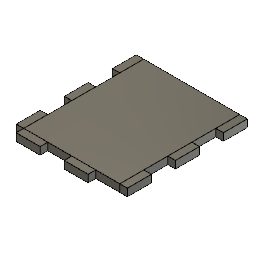
Assembly (Autodesk Fusion 360 archive; units mm, degrees)
design "Top"
Autodesk Fusion 360 part; units mm, degrees
sketch "Sketch1" plane through (0, 0, 0) normal (0, 1, 0) x (1, 0, 0)
  line L0 (0, 0) -> (80, 0)
  line L1 (80, 0) -> (80, 100)
  line L2 (80, 100) -> (0, 100)
  line L3 (0, 100) -> (0, 0)
  line L4 (0, 0) -> (20, 0)
  line L5 (20, 0) -> (20, -6.35)
  line L6 (20, -6.35) -> (0, -6.35)
  line L7 (0, -6.35) -> (0, 0)
  line L8 (40, 0) -> (60, 0)
  line L9 (60, 0) -> (60, -6.35)
  line L10 (60, -6.35) -> (40, -6.35)
  line L11 (40, -6.35) -> (40, 0)
  line L12 (0, 0) -> (-6.35, 0)
  line L13 (-6.35, 0) -> (-6.35, 20)
  line L14 (-6.35, 20) -> (0, 20)
  line L15 (0, 20) -> (0, 0)
  line L16 (0, 40) -> (-6.35, 40)
  line L17 (-6.35, 40) -> (-6.35, 60)
  line L18 (-6.35, 60) -> (0, 60)
  line L19 (0, 60) -> (0, 40)
  line L20 (0, 80) -> (-6.35, 80)
  line L21 (-6.35, 80) -> (-6.35, 100)
  line L22 (-6.35, 100) -> (0, 100)
  line L23 (0, 100) -> (0, 80)
  line L24 (80, 0) -> (86.35, 0)
  line L25 (86.35, 0) -> (86.35, 20)
  line L26 (86.35, 20) -> (80, 20)
  line L27 (80, 20) -> (80, 0)
  line L28 (80, 60) -> (86.35, 60)
  line L29 (86.35, 60) -> (86.35, 40)
  line L30 (86.35, 40) -> (80, 40)
  line L31 (80, 40) -> (80, 60)
  line L32 (80, 100) -> (86.35, 100)
  line L33 (86.35, 100) -> (86.35, 80)
  line L34 (86.35, 80) -> (80, 80)
  line L35 (80, 80) -> (80, 100)
  dimension "d1" = 100
  dimension "d2" = 80
  dimension "d5" = 20
  dimension "d6" = 6.35
  dimension "d7" = 6.35
  dimension "d8" = 20
  dimension "d9" = 20
  dimension "d10" = 6.35
  dimension "d11" = 20
  dimension "d12" = 6.35
  dimension "d13" = 20
  dimension "d14" = 20
  dimension "d15" = 6.35
  dimension "d16" = 20
  dimension "d17" = 20
  dimension "d18" = 6.35
  dimension "d19" = 20
  dimension "d20" = 6.35
  dimension "d21" = 20
  dimension "d22" = 20
  dimension "d23" = 6.35
  dimension "d24" = 20
  measures "d1" distance of L0.start
  measures "d2" distance of L0.start
  measures "d6" distance of L0.start
  measures "d9" distance of L5 L11
  measures "d10" distance of L0.start
  measures "d14" distance of L14 L16
  measures "d17" distance of L18 L20
  measures "d19" distance of L0.start
extrude "Extrude2" add sketch "Sketch1" along normal blind 6.35 makes body 1
extrude "Extrude1" add sketch "Sketch1" along normal blind 6.35 separate body contours L0 L1 L2 L3 L4 L8 L15 L19 L23 L27 L31 L35 makes body 2

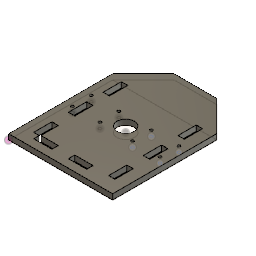
design "Base"
Autodesk Fusion 360 part; units mm, degrees
sketch "Sketch1" plane through (0, 0, 0) normal (0, 1, 0) x (1, 0, 0)
  line L0 (0, 0) -> (120, 0)
  line L1 (120, 0) -> (120, 120)
  line L2 (120, 120) -> (0, 120)
  line L3 (0, 120) -> (0, 0)
  line L4 (0, 120) -> (35.3553, 155.3553)
  line L5 (120, 120) -> (84.6447, 155.3553)
  line L6 (35.3553, 155.3553) -> (84.6447, 155.3553)
  circle A0 centre (60, 75) radius 10
  circle A1 centre (9.5, 64.15) radius 1.65
  circle A2 centre (41.25, 64.15) radius 1.65
  circle A3 centre (41.25, 85.85) radius 1.65
  circle A4 centre (9.5, 85.85) radius 1.65
  circle A5 centre (110.5, 85.85) radius 1.65
  circle A6 centre (110.5, 64.15) radius 1.65
  circle A7 centre (78.75, 64.15) radius 1.65
  circle A8 centre (78.75, 85.85) radius 1.65
  dimension "d1" = 120
  dimension "d2" = 120
  dimension "d3" = 50
  dimension "d4" = 45
  dimension "d5" = 50
  dimension "d6" = 45
  dimension "d7" = 20
  dimension "d8" = 75
  dimension "d9" = 60
  dimension "d10" = 3.3
  dimension "d11" = 3.3
  dimension "d12" = 9.5
  dimension "d13" = 31.75
  dimension "d14" = 10.85
  dimension "d15" = 10.85
  dimension "d16" = 3.3
  dimension "d17" = 3.3
  dimension "d18" = 21.7
  dimension "d19" = 21.7
  dimension "d20" = 9.5
  dimension "d21" = 31.75
  dimension "d22" = 3.3
  dimension "d23" = 3.3
  dimension "d24" = 31.75
  dimension "d25" = 3.3
  dimension "d26" = 3.3
  dimension "d27" = 21.7
  dimension "d28" = 21.7
  dimension "d29" = 31.75
  dimension "d30" = 9.5
  measures "d4" angle of L2 L4
  measures "d6" angle of L2 L5
  measures "d7" diameter of A0
  measures "d10" diameter of A1
  measures "d11" diameter of A2
  measures "d13" distance of L0.start
  measures "d15" distance of L0.start
  measures "d16" diameter of A3
  measures "d17" diameter of A4
  measures "d21" distance of L0.start
  measures "d22" diameter of A7
  measures "d23" diameter of A6
  measures "d25" diameter of A5
  measures "d26" diameter of A8
extrude "Extrude1" add sketch "Sketch1" along normal blind 6.35
sketch "Sketch2" plane through (0, 6.35, 0) normal (0, 1, 0) x (-1, 0, 0)
  circle A0 centre (-78.75, -64.15) radius 1.65
  circle A1 centre (-78.75, -85.85) radius 1.65
  circle A2 centre (-41.25, -85.85) radius 1.65
  circle A3 centre (-9.5, -85.85) radius 1.65
  circle A4 centre (-110.5, -85.85) radius 1.65
  circle A5 centre (-41.25, -64.15) radius 1.65
  circle A6 centre (-9.5, -64.15) radius 1.65
  circle A7 centre (-60, -75) radius 10
  circle A8 centre (-110.5, -64.15) radius 1.65
  line L0 (0, -120) -> (0, 0)
  line L1 (0, 0) -> (-120, 0)
  line L2 (-120, 0) -> (-120, -120)
  line L3 (-120, -120) -> (-84.6447, -155.3553)
  line L4 (-84.6447, -155.3553) -> (-35.3553, -155.3553)
  line L5 (-35.3553, -155.3553) -> (0, -120)
  line L6 (-20, -16.35) -> (-40, -16.35)
  line L7 (-40, -16.35) -> (-40, -10)
  line L8 (-40, -10) -> (-20, -10)
  line L9 (-20, -10) -> (-20, -16.35)
  line L10 (0, 0) -> (-120, 0)
  line L11 (0, -120) -> (0, 0)
  line L12 (-60, -16.35) -> (-80, -16.35)
  line L13 (-80, -16.35) -> (-80, -10)
  line L14 (-80, -10) -> (-60, -10)
  line L15 (-60, -10) -> (-60, -16.35)
  line L16 (-20, -16.35) -> (-13.65, -16.35)
  line L17 (-13.65, -16.35) -> (-13.65, -36.35)
  line L18 (-13.65, -36.35) -> (-20, -36.35)
  line L19 (-20, -36.35) -> (-20, -16.35)
  line L20 (-13.65, -56.35) -> (-20, -56.35)
  line L21 (-20, -56.35) -> (-20, -76.35)
  line L22 (-20, -76.35) -> (-13.65, -76.35)
  line L23 (-13.65, -76.35) -> (-13.65, -56.35)
  line L24 (-20, -96.35) -> (-13.65, -96.35)
  line L25 (-13.65, -96.35) -> (-13.65, -116.35)
  line L26 (-13.65, -116.35) -> (-20, -116.35)
  line L27 (-20, -116.35) -> (-20, -96.35)
  line L28 (-106.35, -16.35) -> (-100, -16.35)
  line L29 (-100, -16.35) -> (-100, -36.35)
  line L30 (-100, -36.35) -> (-106.35, -36.35)
  line L31 (-106.35, -36.35) -> (-106.35, -16.35)
  line L32 (-120, 0) -> (-120, -120)
  line L33 (-100, -76.35) -> (-106.35, -76.35)
  line L34 (-106.35, -76.35) -> (-106.35, -56.35)
  line L35 (-106.35, -56.35) -> (-100, -56.35)
  line L36 (-100, -56.35) -> (-100, -76.35)
  line L37 (-100, -96.35) -> (-106.35, -96.35)
  line L38 (-106.35, -96.35) -> (-106.35, -116.35)
  line L39 (-106.35, -116.35) -> (-100, -116.35)
  line L40 (-100, -116.35) -> (-100, -96.35)
  line L41 (-99.5, -116.85) -> (-99.5, -95.85)
  line L42 (-99.5, -95.85) -> (-106.85, -95.85)
  line L43 (-106.85, -95.85) -> (-106.85, -116.85)
  line L44 (-106.85, -116.85) -> (-99.5, -116.85)
  line L45 (-99.5, -55.85) -> (-99.5, -76.85)
  line L46 (-99.5, -76.85) -> (-106.85, -76.85)
  line L47 (-106.85, -76.85) -> (-106.85, -55.85)
  line L48 (-106.85, -55.85) -> (-99.5, -55.85)
  line L49 (-99.5, -15.85) -> (-99.5, -36.85)
  line L50 (-99.5, -36.85) -> (-106.85, -36.85)
  line L51 (-106.85, -36.85) -> (-106.85, -15.85)
  line L52 (-106.85, -15.85) -> (-99.5, -15.85)
  line L53 (-59.5, -16.85) -> (-80.5, -16.85)
  line L54 (-80.5, -16.85) -> (-80.5, -9.5)
  line L55 (-80.5, -9.5) -> (-59.5, -9.5)
  line L56 (-59.5, -9.5) -> (-59.5, -16.85)
  line L57 (-19.5, -16.85) -> (-40.5, -16.85)
  line L58 (-40.5, -16.85) -> (-40.5, -9.5)
  line L59 (-40.5, -9.5) -> (-19.5, -9.5)
  line L60 (-19.5, -9.5) -> (-19.5, -16.85)
  line L61 (-20.5, -15.85) -> (-13.15, -15.85)
  line L62 (-13.15, -15.85) -> (-13.15, -36.85)
  line L63 (-13.15, -36.85) -> (-20.5, -36.85)
  line L64 (-20.5, -36.85) -> (-20.5, -15.85)
  line L65 (-20.5, -55.85) -> (-20.5, -76.85)
  line L66 (-20.5, -76.85) -> (-13.15, -76.85)
  line L67 (-13.15, -76.85) -> (-13.15, -55.85)
  line L68 (-13.15, -55.85) -> (-20.5, -55.85)
  line L69 (-13.15, -116.85) -> (-20.5, -116.85)
  line L70 (-20.5, -116.85) -> (-20.5, -95.85)
  line L71 (-20.5, -95.85) -> (-13.15, -95.85)
  line L72 (-13.15, -95.85) -> (-13.15, -116.85)
  dimension "d33" = 6.35
  dimension "d34" = 20
  dimension "d35" = 10
  dimension "d37" = 6.35
  dimension "d38" = 20
  dimension "d39" = 20
  dimension "d40" = 10
  dimension "d41" = 20
  dimension "d42" = 6.35
  dimension "d43" = 20
  dimension "d44" = 6.35
  dimension "d45" = 20
  dimension "d48" = 20
  dimension "d49" = 6.35
  dimension "d51" = 20
  dimension "d52" = 20
  dimension "d53" = 6.35
  dimension "d55" = 16.35
  dimension "d56" = 20
  dimension "d57" = 20
  dimension "d58" = 20
  dimension "d59" = 20
  dimension "d60" = 20
  dimension "d61" = 6.35
  dimension "d62" = 20
  dimension "d63" = 20
  dimension "d64" = 20
  dimension "d65" = 6.35
  dimension "d66" = 20
  dimension "d67" = 20
  dimension "d68" = 0.5
  dimension "d69" = -0.5
  dimension "d70" = -0.5
  dimension "d71" = -0.5
  dimension "d72" = -0.5
  dimension "d73" = -0.5
  dimension "d74" = 0.5
  dimension "d75" = -0.5
  measures "d35" distance of L8 L10
  measures "d39" distance of L7 L15
  measures "d40" distance of L10 L14
  measures "d41" distance of L0.end
  measures "d42" distance of L0.end
  measures "d44" distance of L0.end
  measures "d45" distance of L18 L20
  measures "d49" distance of L0.end
  measures "d51" distance of L22 L24
  measures "d52" distance of L0.end
  measures "d55" distance of L10 L28
  measures "d56" distance of L29 L32
  measures "d57" distance of L11 L19
  measures "d58" distance of L11 L21
  measures "d59" distance of L11 L27
  measures "d62" distance of L32 L36
  measures "d63" distance of L30 L35
  measures "d66" distance of L32 L40
  measures "d67" distance of L33 L37
  measures "d70" distance of L29
  measures "d71" distance of L12
  measures "d72" distance of L6
  measures "d73" distance of L16
  measures "d75" distance of L26
extrude "Extrude2" cut sketch "Sketch2" against normal blind 6.35 contours L6 L19 L57 L64 | L6 L9 L61 L64 | L9 L16 L60 L61 | L16 L19 L57 L60 | L6 L7 L8 L9 L57 L58 L59 L60 L61 L64 | L6 L7 L8 L9 L61 L64 | L16 L17 L18 L19 L57 L60 L61 L62 L63 L64 | L16 L17 L18 L19 L57 L60 | L12 L13 L14 L15 | L20 L21 L22 L23 | L24 L25 L26 L27 | L28 L29 L30 L31 | L33 L34 L35 L36 | L37 L38 L39 L40 | L41 L42 L43 L44 | L45 L46 L47 L48 | L49 L50 L51 L52 | L53 L54 L55 L56 | L65 L66 L67 L68 | L69 L70 L71 L72

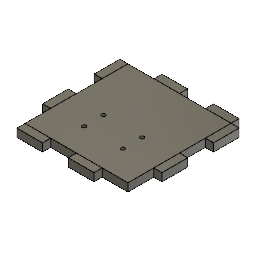
design "Front"
Autodesk Fusion 360 part; units mm, degrees
sketch "Sketch1" plane through (0, 0, 0) normal (0, 1, 0) x (1, 0, 0)
  line L0 (0, 0) -> (80, 0)
  line L1 (80, 0) -> (80, 80)
  line L2 (80, 80) -> (0, 80)
  line L3 (0, 80) -> (0, 0)
  circle A0 centre (25, 21) radius 1.5
  circle A1 centre (25, 36) radius 1.5
  circle A2 centre (55, 21) radius 1.5
  circle A3 centre (55, 36) radius 1.5
  line L4 (0, 0) -> (20, 0)
  line L5 (20, 0) -> (20, -6.35)
  line L6 (20, -6.35) -> (0, -6.35)
  line L7 (0, -6.35) -> (0, 0)
  line L8 (40, 0) -> (60, 0)
  line L9 (60, 0) -> (60, -6.35)
  line L10 (60, -6.35) -> (40, -6.35)
  line L11 (40, -6.35) -> (40, 0)
  line L12 (80, 20) -> (86.35, 20)
  line L13 (86.35, 20) -> (86.35, 40)
  line L14 (86.35, 40) -> (80, 40)
  line L15 (80, 40) -> (80, 20)
  line L16 (80, 60) -> (86.35, 60)
  line L17 (86.35, 60) -> (86.35, 80)
  line L18 (86.35, 80) -> (80, 80)
  line L19 (80, 80) -> (80, 60)
  line L20 (0, 20) -> (-6.35, 20)
  line L21 (-6.35, 20) -> (-6.35, 40)
  line L22 (-6.35, 40) -> (0, 40)
  line L23 (0, 40) -> (0, 20)
  line L24 (0, 60) -> (-6.35, 60)
  line L25 (-6.35, 60) -> (-6.35, 80)
  line L26 (-6.35, 80) -> (0, 80)
  line L27 (0, 80) -> (0, 60)
  line L28 (80, 80) -> (60, 80)
  line L29 (60, 80) -> (60, 86.35)
  line L30 (60, 86.35) -> (80, 86.35)
  line L31 (80, 86.35) -> (80, 80)
  line L32 (40, 80) -> (20, 80)
  line L33 (20, 80) -> (20, 86.35)
  line L34 (20, 86.35) -> (40, 86.35)
  line L35 (40, 86.35) -> (40, 80)
  dimension "d1" = 80
  dimension "d2" = 80
  dimension "d3" = 3
  dimension "d4" = 3
  dimension "d5" = 3
  dimension "d6" = 3
  dimension "d7" = 21
  dimension "d8" = 15
  dimension "d9" = 21
  dimension "d10" = 15
  dimension "d11" = 30
  dimension "d12" = 30
  dimension "d13" = 25
  dimension "d19" = 6.35
  dimension "d20" = 20
  dimension "d21" = 6.35
  dimension "d22" = 20
  dimension "d23" = 20
  dimension "d24" = 6.35
  dimension "d25" = 20
  dimension "d26" = 20
  dimension "d27" = 20
  dimension "d28" = 6.35
  dimension "d29" = 20
  dimension "d30" = 6.35
  dimension "d31" = 20
  dimension "d32" = 6.35
  dimension "d33" = 20
  dimension "d34" = 20
  dimension "d35" = 20
  dimension "d36" = 6.35
  dimension "d37" = 20
  dimension "d38" = 6.35
  dimension "d39" = 20
  dimension "d40" = 20
  measures "d1" distance of L0.start
  measures "d3" diameter of A0
  measures "d4" diameter of A1
  measures "d5" diameter of A2
  measures "d6" diameter of A3
  measures "d19" distance of L0.start
  measures "d21" distance of L0.start
  measures "d23" distance of L5 L11
  measures "d25" distance of L0 L12
  measures "d29" distance of L14 L16
  measures "d34" distance of L22 L24
  measures "d35" distance of L0 L20
  measures "d40" distance of L29 L35
extrude "Extrude2" add sketch "Sketch1" along normal blind 6.35 makes body 1
extrude "Extrude1" add sketch "Sketch1" along normal blind 6.35 separate body contours L0 L1 L2 L3 L4 L8 L15 L19 L23 L27 L28 L32 makes body 2
equation "height = 75 mm" comment "Height of the front"
equation "Acryllic_thickness = 6.35 mm"

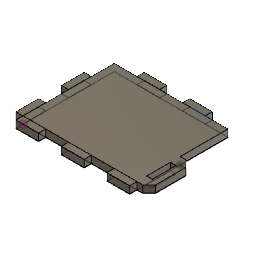
design "Right Side"
Autodesk Fusion 360 part; units mm, degrees
sketch "Sketch1" plane through (0, 0, 0) normal (0, 1, 0) x (1, 0, 0)
  line L0 (0, 0) -> (100, 0)
  line L1 (100, 0) -> (100, 80)
  line L2 (100, 80) -> (0, 80)
  line L3 (0, 80) -> (0, 0)
  line L4 (100, 29.5) -> (105, 29.5)
  line L5 (105, 29.5) -> (105, 8.5)
  line L6 (105, 8.5) -> (100, 8.5)
  line L7 (100, 8.5) -> (100, 29.5)
  line L8 (100, 0) -> (105, 0)
  line L9 (105, 0) -> (110.6569, 5.6569)
  line L10 (100, 38) -> (105, 38)
  line L11 (105, 38) -> (110.6569, 32.3431)
  line L12 (110.6569, 32.3431) -> (110.6569, 5.6569)
  line L13 (0, 0) -> (20, 0)
  line L14 (20, 0) -> (20, -6.35)
  line L15 (20, -6.35) -> (0, -6.35)
  line L16 (0, -6.35) -> (0, 0)
  line L17 (40, 0) -> (60, 0)
  line L18 (60, 0) -> (60, -6.35)
  line L19 (60, -6.35) -> (40, -6.35)
  line L20 (40, -6.35) -> (40, 0)
  line L21 (80, 0) -> (100, 0)
  line L22 (100, 0) -> (100, -6.35)
  line L23 (100, -6.35) -> (80, -6.35)
  line L24 (80, -6.35) -> (80, 0)
  line L25 (0, 0) -> (-6.35, 0)
  line L26 (-6.35, 0) -> (-6.35, 20)
  line L27 (-6.35, 20) -> (0, 20)
  line L28 (0, 20) -> (0, 0)
  line L29 (0, 40) -> (-6.35, 40)
  line L30 (-6.35, 40) -> (-6.35, 60)
  line L31 (-6.35, 60) -> (0, 60)
  line L32 (0, 60) -> (0, 40)
  line L33 (20, 80) -> (40, 80)
  line L34 (40, 80) -> (40, 86.35)
  line L35 (40, 86.35) -> (20, 86.35)
  line L36 (20, 86.35) -> (20, 80)
  line L37 (60, 80) -> (80, 80)
  line L38 (80, 80) -> (80, 86.35)
  line L39 (80, 86.35) -> (60, 86.35)
  line L40 (60, 86.35) -> (60, 80)
  dimension "d1" = 80
  dimension "d2" = 100
  dimension "d3" = 5
  dimension "d4" = 21
  dimension "d6" = 8.5
  dimension "d7" = 5
  dimension "d8" = 8
  dimension "d10" = 45
  dimension "d11" = 5
  dimension "d12" = 8.5
  dimension "d13" = 8
  dimension "d14" = 45
  dimension "d17" = 20
  dimension "d18" = 6.35
  dimension "d19" = 6.35
  dimension "d20" = 20
  dimension "d21" = 40
  dimension "d22" = 6.35
  dimension "d23" = 20
  dimension "d24" = 20
  dimension "d25" = 6.35
  dimension "d26" = 20
  dimension "d27" = 6.35
  dimension "d28" = 20
  dimension "d29" = 20
  dimension "d32" = 6.35
  dimension "d33" = 20
  dimension "d34" = 6.35
  dimension "d35" = 20
  dimension "d36" = 20
  dimension "d37" = 20
  measures "d1" distance of L0.start
  measures "d2" distance of L0.start
  measures "d4" distance of L0.start
  measures "d6" distance of L0 L6
  measures "d7" distance of L0.start
  measures "d8" distance of L0.start
  measures "d10" angle of L5 L9
  measures "d12" distance of L4 L10
  measures "d14" angle of L5 L11
  measures "d18" distance of L0.start
  measures "d19" distance of L0.start
  measures "d21" distance of L16 L20
  measures "d24" distance of L18 L24
  measures "d25" distance of L0.start
  measures "d27" distance of L13.end
  measures "d28" distance of L29 L31
  measures "d29" distance of L27 L29
  measures "d36" distance of L34 L40
  measures "d37" distance of L3 L36
extrude "Extrude3" add sketch "Sketch1" along normal blind 6.35 contours L0 L1 L2 L3 L7 L13 L17 L21 L28 L32 L33 L37 | L3 L25 L26 L27 L28 | L0 L13 L14 L15 L16 | L0 L17 L18 L19 L20 | L3 L29 L30 L31 L32 | L0 L21 L22 L23 L24 | L1 L4 L5 L6 L8 L9 L10 L11 L12 | L2 L33 L34 L35 L36 | L2 L37 L38 L39 L40 makes body 1
extrude "Extrude2" add sketch "Sketch1" along normal blind 6.35 separate body contours L0 L1 L2 L3 L7 L13 L17 L21 L28 L32 L33 L37 | L3 L25 L26 L27 L28 | L0 L13 L14 L15 L16 | L0 L17 L18 L19 L20 | L3 L29 L30 L31 L32 | L0 L21 L22 L23 L24 | L1 L4 L5 L6 L8 L9 L10 L11 L12 makes body 2
extrude "Extrude1" add sketch "Sketch1" along normal blind 6.35 separate body contours L0 L1 L2 L3 L7 L13 L17 L21 L28 L32 L33 L37 | L1 L4 L5 L6 L8 L9 L10 L11 L12 makes body 3
equation "d6 = ( 17 / 2 ) * 1 mm"
equation "d12 = ( 17 / 2 ) * 1 mm"
